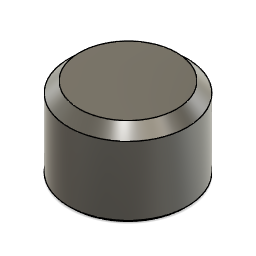
RotEncKnob (Autodesk Fusion 360 design; units mm, degrees)
Autodesk Fusion 360 part; units mm, degrees
sketch "Skizze1" plane through (0, 0, 0) normal (0, 1, 0) x (1, 0, 0)
  circle A0 centre (0, 0) radius 8.75
  circle A1 centre (0, 0) radius 11.25
  dimension "d1" = 17.5
  dimension "d3" = 2.5
  constraint coincident A0.centre A1.centre
  constraint concentric A0 A1
  measures "d1" diameter of A0
  measures "d3" distance of A0 A1
extrude "Extrusion1" add sketch "Skizze1" along normal blind 13
sketch "Skizze3" plane through (0, 13, 0) normal (0, 1, 0) x (-1, 0, 0)
  circle A0 centre (0, 0) radius 8.75
  circle A1 centre (0, 0) radius 11.25
extrude "Extrusion2" add sketch "Skizze3" along normal blind 2.5 contours A0 | A1
sketch "Skizze4" plane through (0, 13, 0) normal (0, -1, 0) x (1, 0, 0)
  circle A0 centre (0, 0) radius 8.75
  circle A1 centre (0, 0) radius 3.32
  circle A2 centre (0, 0) radius 5.82
  line L0 (-2.936, 1.55) -> (2.936, 1.55)
  line L1 (0, 0) -> (0, -11.7382) construction
  point P0 (0, -3.32)
  dimension "d11" = 6.64
  dimension "d12" = 2.5
  dimension "d13" = 4.87
  constraint coincident A0.centre A1.centre
  constraint concentric A1 A2
  constraint coincident A1 L0.start
  constraint coincident A1 L0.end
  constraint horizontal L0
  constraint vertical L1
  constraint coincident A1 P0
  constraint coincident L1 P0
  measures "d11" diameter of A1
  measures "d12" distance of A1 A2
  measures "d13" distance of L0 P0
extrude "Extrusion3" add sketch "Skizze4" along normal blind 9.68 contours A1 L0 | A2 picked at (0.7906, 1.8078)
chamfer "Fase1" distance 2 angle 45 1 edges at (10.4887, 15.5, -4.0682)
chamfer "Fase2" distance 0.5 angle 45 1 edges at (-8.1579, 13, -3.1641)
chamfer "Fase3" distance 0.5 angle 45 1 edges at (-5.4261, 13, 2.1046)
chamfer "Fase4" distance 0.5 angle 45 1 edges at (-5.4261, 3.32, -2.1046)
chamfer "Fase5" distance 0.8 angle 45 2 edges at (0, 3.32, -3.32) (0, 3.32, 1.55)
chamfer "Fase6" distance 0.5 angle 45 2 edges at (-8.1579, 0, -3.1641) (-10.4887, 0, 4.0682)
equation "d1 = 20 mm - wall_thickness"
equation "wall_thickness = 2.5 mm"
equation "d3 = wall_thickness"
equation "pin_height = 15 mm"
equation "knob_plate_distance = 2 mm"
equation "d6 = pin_height - knob_plate_distance"
equation "d8 = wall_thickness"
equation "clearance = 0.32 mm"
equation "d11 = 6 mm + 2 * clearance"
equation "d12 = wall_thickness"
equation "d13 = 4.55 mm + clearance"
equation "d14 = 10 mm - clearance"
